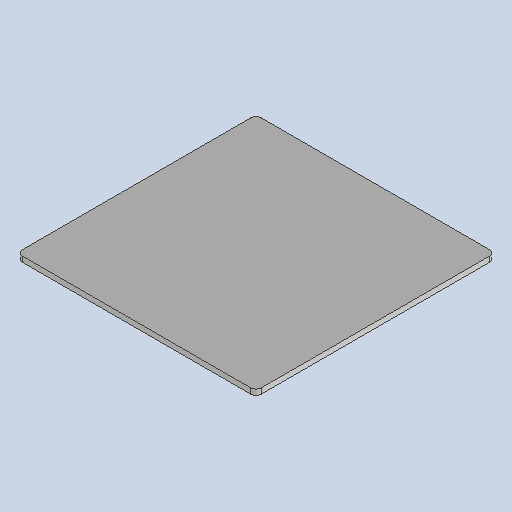
# Autodesk Inventor part: PRS 1665 DrSysB CUP 1_1200
Saved by Autodesk Inventor 2026.2 (Build 302298000, 298)
## iProperties
Created: 2025-06-24
Part Number: PRS 1665 DrSysB CUP 1_1200
Material: Stainless Steel
Document SubType Name: Sheet Metal
Designer: admin
Mass: 118.281 g
Surface Area: 154.663 cm^2
Volume: 14.7851 cm^3
Density: 8 g/cm^3
Flat Pattern Width: 8.8 cm
Flat Pattern Length: 8.8 cm
Flat Pattern Area: 77.44 cm^2
Sheet Metal Rule: AISI304 2mm Die16
Sheet Metal Width: 88,000 mm
Sheet Metal Length: 88,000 mm
Sheet Metal Area: 7744,000 mm^2
Appearance: Default
Author: user
Autodesk Inventor part; units mm, degrees
ref_plane "YZ Plane" through (0, 0, 0) normal (1, 0, 0) x (0, 1, 0)
ref_plane "XZ Plane" through (0, 0, 0) normal (0, 1, 0) x (-1, 0, 0)
ref_plane "XY Plane" through (0, 0, 0) normal (0, 0, 1) x (1, 0, 0)
sketch "Sketch1" plane through (0, 0, 0) normal (0, 0, 1) x (1, 0, 0)
  line L0 (-44, -44) -> (44, -44)
  line L1 (44, -44) -> (44, 44)
  line L2 (44, 44) -> (-44, 44)
  line L3 (-44, 44) -> (-44, -44)
  line L4 (-44, -44) -> (44, 44) construction
  line L5 (44, -44) -> (-44, 44) construction
  point P0 (0, 0)
  dimension "d154" = 88
  dimension "d155" = 88
  measures "d154" distance of L1.end L2.end
  measures "d155" distance of L0.end L1.end
extrude "Plate5" add sketch "Sketch1" along normal blind 2
fillet "Corner Round1" radius 2 4 edges at (44, 44, 1) (-44, 44, 1) (-44, -44, 1) (44, -44, 1)
body "Solid3"
